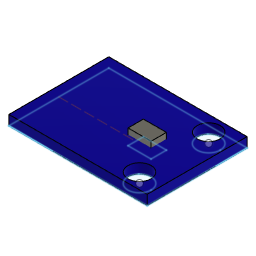
tsl2561 (Autodesk Fusion 360 design; units mm, degrees)
Autodesk Fusion 360 part; units mm, degrees
sketch "Esquisse1" plane through (0, 0, 0) normal (0, 0, 1) x (1, 0, 0)
  line L0 (0, 13) -> (18, 13)
  line L1 (18, 13) -> (18, 0)
  line L2 (18, 0) -> (0, 0)
  line L3 (0, 0) -> (0, 13)
  circle A0 centre (15, 11) radius 1.5
  circle A1 centre (15, 2) radius 1.5
  line L4 (10, 7.5) -> (13, 7.5)
  line L5 (13, 7.5) -> (13, 5.5)
  line L6 (13, 5.5) -> (10, 5.5)
  line L7 (10, 5.5) -> (10, 7.5)
  line L8 (0, 6.5) -> (10, 6.5) construction
  dimension "d1" = 18
  dimension "d2" = 13
  dimension "d5" = 3
  dimension "d6" = 3
  constraint horizontal L0
  constraint vertical L1
  constraint horizontal L2
  constraint vertical L3
  constraint horizontal L4
  constraint vertical L5
  constraint horizontal L6
  constraint vertical L7
  constraint midpoint L3 L8.start
  constraint coincident L7 L8.end
  constraint perpendicular L7 L8
  measures "d1" distance of L0.start L0.end
  measures "d2" distance of L0.start L2.end
  measures "d5" diameter of A0
  measures "d6" diameter of A1
extrude "Extrusion2" add sketch "Esquisse1" along normal blind 2 contours L4 L5 L6 L7 makes body 1
extrude "Extrusion1" add sketch "Esquisse1" along normal blind 1.27 separate body contours L0 L1 L2 L3 | L4 L5 L6 L7 makes body 2
